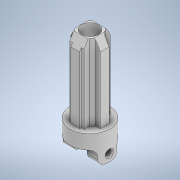
# Autodesk Inventor part: upper plug
Saved by Autodesk Inventor 2022 (Build 260153000, 153)
## iProperties
Created: 2022-03-20
Part Number: upper plug
Material: Generic
Document SubType Name: Modeling
Designer: Dahway
Density: 1 g/cm^3
Appearance: Default
Author: Dahway
Autodesk Inventor part; units mm, degrees
ref_plane "YZ Plane" through (0, 0, 0) normal (1, 0, 0) x (0, 1, 0)
ref_plane "XZ Plane" through (0, 0, 0) normal (0, 1, 0) x (-1, 0, 0)
ref_plane "XY Plane" through (0, 0, 0) normal (0, 0, 1) x (1, 0, 0)
sketch "Sketch1" plane through (0, 0, 0) normal (0, 1, 0) x (-1, 0, 0)
  circle A0 centre (0, 0) radius 7
  dimension "d0" = 14
  constraints: 1 centre point, 1 coincident
  measures "d0" diameter of A0
extrude "Extrusion1" add sketch "Sketch1" along normal blind 5
sketch "Sketch2" plane through (0, 5, 0) normal (0, 1, 0) x (1, 0, 0)
  circle A0 centre (0, 0) radius 3.8
  circle A1 centre (0, 0) radius 7 projected
  line L0 (-1.55, 5.2) -> (1.55, 5.2)
  line L1 (1.55, 5.2) -> (1.55, 2.4)
  line L2 (1.55, 2.4) -> (-1.55, 2.4)
  line L3 (-1.55, 2.4) -> (-1.55, 5.2)
  line L4 (-1.55, 5.2) -> (1.55, 2.4) construction
  line L5 (1.55, 5.2) -> (-1.55, 2.4) construction
  circle A2 centre (0, 0) radius 3.8
  line L6 (-5.2, -1.55) -> (-5.2, 1.55)
  line L7 (-5.2, 1.55) -> (-2.4, 1.55)
  line L8 (-2.4, 1.55) -> (-2.4, -1.55)
  line L9 (-2.4, -1.55) -> (-5.2, -1.55)
  line L10 (-5.2, -1.55) -> (-2.4, 1.55) construction
  line L11 (-5.2, 1.55) -> (-2.4, -1.55) construction
  circle A3 centre (0, 0) radius 3.8
  line L12 (1.55, -5.2) -> (-1.55, -5.2)
  line L13 (-1.55, -5.2) -> (-1.55, -2.4)
  line L14 (-1.55, -2.4) -> (1.55, -2.4)
  line L15 (1.55, -2.4) -> (1.55, -5.2)
  line L16 (1.55, -5.2) -> (-1.55, -2.4) construction
  line L17 (-1.55, -5.2) -> (1.55, -2.4) construction
  circle A4 centre (0, 0) radius 3.8
  line L18 (5.2, 1.55) -> (5.2, -1.55)
  line L19 (5.2, -1.55) -> (2.4, -1.55)
  line L20 (2.4, -1.55) -> (2.4, 1.55)
  line L21 (2.4, 1.55) -> (5.2, 1.55)
  line L22 (5.2, 1.55) -> (2.4, -1.55) construction
  line L23 (5.2, -1.55) -> (2.4, 1.55) construction
  line L24 (2.55, 4.6) -> (-2.55, 4.6)
  line L25 (-2.55, 4.6) -> (-2.55, 2.8174)
  line L26 (-2.55, 2.8174) -> (2.55, 2.8174)
  line L27 (2.55, 2.8174) -> (2.55, 4.6)
  line L28 (-2.55, -2.8174) -> (-2.55, -4.6)
  line L29 (-2.55, -4.6) -> (2.55, -4.6)
  line L30 (2.55, -4.6) -> (2.55, -2.8174)
  point P0 (0, 3.8)
  point P1 (-3.8, 0)
  point P2 (0, -3.8)
  point P3 (3.8, 0)
  point P4 (-1.55, 3.4695)
  point P5 (-3.4695, 1.55)
  point P6 (-3.4695, -1.55)
  point P7 (-1.55, -3.4695)
  point P8 (1.55, -3.4695)
  point P9 (3.4695, -1.55)
  point P10 (3.4695, 1.55)
  point P11 (1.55, 3.4695)
  point P12 (2.55, -2.8174)
  point P13 (1.55, -4.6)
  point P14 (-1.55, -4.6)
  point P15 (-2.55, -2.8174)
  point P16 (-2.55, 2.8174)
  point P17 (-1.55, 4.6)
  point P18 (2.55, 2.8174)
  point P19 (1.55, 4.6)
  dimension "d65" = 7.6
  dimension "d66" = 3.2
  dimension "d67" = 3.1
  dimension "d68" = 2.8
  dimension "d71" = 360
  dimension "d75" = 5.1
  dimension "d76" = 0.6
  dimension "d80" = 360
  dimension "d88" = 2.55
  dimension "d89" = 2.4
  constraints: 62 end point, 8 midpoint, 4 coincident, 4 parallel, 2 coincident with centre, 2 horizontal, 2 perpendicular, 2 point on circle, 1 centre point, 1 horizontal alignment, 1 vertical alignment, 71 other
  measures "d67" distance of L1.end L2.end
  measures "d68" distance of L0.end L1.end
  measures "d75" distance of L26.end L25.end
  measures "d76" distance between parallel lines of L24 L0
  measures "d88" distance from line of point (0, 0) L27
  measures "d89" distance from line of point (0, 0) L2
extrude "Extrusion2" add sketch "Sketch2" along normal blind 27 contours A0 L19 L20 L21 | A0 L21 L18 L19 | L21 L20 L19 A0 L15 L14 L13 L9 L8 L7 L26 L3 L2 L1 | L26 L1 A0 | A0 L1 L24 L27 | L30 L29 L15 A0 | L1 L26 L3 A0 | A0 L3 L24 L1 | L1 L2 L3 L26 | L15 L29 L13 A0 | A0 L13 L14 L15 | L3 L26 A0 | A0 L25 L24 L3 | L24 L3 L0 L1 | L13 L29 L28 A0 | L15 L12 L13 L29 | L7 L8 L9 A0 | A0 L9 L6 L7
sketch "Sketch3" plane through (0, 32, 0) normal (0, 1, 0) x (1, 0, 0)
  line L0 (-5.25, -1.5) -> (-3.4369, -1.5) projected
  line L1 (3.4369, -1.5) -> (5.25, -1.5) projected
  circle A0 centre (0, 0) radius 3
  point P0 (0, 0)
  dimension "d61" = 6
  constraints: 1 centre point, 1 coincident
  measures "d61" diameter of A0
extrude "Extrusion3" cut sketch "Sketch3" against normal blind 7
sketch "Sketch4" plane through (0, 5, 0) normal (0, 1, 0) x (1, 0, 0)
  circle A0 centre (0, 0) radius 7 projected
  line L0 (0, 0) -> (7, 0) construction
  line L1 (0, 0) -> (7, 0) construction
  circle A1 centre (-4.9497, 4.9497) radius 1
  circle A2 centre (-4.9497, -4.9497) radius 1
  circle A3 centre (4.9497, -4.9497) radius 1
  circle A4 centre (4.9497, 4.9497) radius 1
  point P0 (-4.9497, -4.9497)
  point P1 (4.9497, 4.9497)
  point P2 (4.1939, 5.6045)
  point P3 (5.6045, 4.1939)
  point P4 (5.6045, -4.1939)
  point P5 (4.1939, -5.6045)
  point P6 (-5.6045, -4.1939)
  point P7 (-4.1939, -5.6045)
  point P8 (-4.1939, 5.6045)
  point P9 (-5.6045, 4.1939)
  dimension "d26" = 2
  dimension "d29" = 360
  constraints: 4 centre point, 4 end point, 2 horizontal, 2 point on circle, 1 coincident, 9 other
  measures "d26" diameter of A1
extrude "Extrusion4" add sketch "Sketch4" along normal blind 2 contours A4 A0 | A0 A3 | A1 A0 | A0 A2 picked at (4.7103, 4.7103) picked at (4.7103, -4.7103) picked at (-4.6879, 4.735) picked at (-4.6879, -4.735)
sketch "Sketch5" plane through (0, 0, 0) normal (0, -1, 0) x (1, 0, 0)
  line L0 (2.5, 3.45) -> (2.5, -3.45)
  arc A0 (5.6045, -4.1939) -> (5.6045, 4.1939) centre (0, 0) ccw projected
  arc A1 (6.0908, -3.45) -> (6.0908, 3.45) centre (0, 0) ccw
  line L1 (2.5, 3.45) -> (6.0908, 3.45)
  line L2 (2.5, -3.45) -> (6.0908, -3.45)
  dimension "d33" = 6.9
  dimension "d50" = 4.5
  constraints: 6 end point, 4 point on circle, 2 parallel, 1 centre point, 1 horizontal, 1 vertical
  measures "d33" distance of L0.start L0.end
  measures "d50" distance edge to line of A0 L0
extrude "Extrusion5" add sketch "Sketch5" along normal blind 5
pattern_circular "Circular Pattern1" count 2 over 360 about axis through (0, 0, 0) along (0, 1, 0) of "Extrusion5"
fillet "Fillet2" radius 2 10 edges at (4.2954, -5, -3.45) (4.2954, -5, 3.45) (-4.2954, -5, -3.45) (-4.2954, -5, 3.45) (4.2954, 0, -3.45) (-4.2954, 0, -3.45) (-4.2954, 0, 3.45) (4.2954, 0, 3.45) (2.5, 0, 0) (-2.5, 0, 0)
sketch "Sketch7" plane through (2.5, -3, -3.45) normal (-1, 0, 0) x (0, 0, 1)
  line L0 (4.9, -2) -> (2, -2) projected
  line L1 (0, 1) -> (0, 0) projected
  point P0 (3.45, 3)
  point P1 (3.45, 0.5)
  dimension "d52" = 2.5
  dimension "d53" = 3.45
  measures "d52" distance from line of L0 point (3.45, 0.5)
  measures "d53" distance from line of point (3.45, 0.5) L1
hole "Hole2" at (2.5, -2.5, 0) direction (1, 0, 0) diameter 2 end through all both
chamfer "Chamfer2" distance 0.5 angle 45 8 edges at (6.9282, -2.5039, -1) (-6.9282, -2.5039, -1) (2.5, -2.2412, 0.9659) (2.5, -3.4659, -0.2588) (2.4365, -1.5, 0) (-2.5, -3.4659, -0.2588) (-2.5, -2.2412, 0.9659) (-2.4365, -1.5, 0)
chamfer "Chamfer3" distance 2 angle 60 4 edges at (5.2, 32, 0) (0, 32, -5.2) (-5.2, 32, 0) (0, 32, 5.2) measured on face at (0, 32, 4.7) measured on face at (0, 32, -4.7) measured on face at (-4.7, 32, 0) measured on face at (4.7, 32, 0)
sketch "Sketch9" plane through (0, 5, 0) normal (0, 1, 0) x (1, 0, 0)
  arc A0 (-4.1939, -5.6045) -> (-5.6045, -4.1939) centre (-4.9497, -4.9497) ccw projected
  circle A1 centre (-4.9497, -4.9497) radius 1
  arc A2 (5.6045, -4.1939) -> (4.1939, -5.6045) centre (4.9497, -4.9497) ccw projected
  circle A3 centre (4.9497, -4.9497) radius 1
  arc A4 (4.1939, 5.6045) -> (5.6045, 4.1939) centre (4.9497, 4.9497) ccw projected
  circle A5 centre (4.9497, 4.9497) radius 1
  circle A6 centre (-4.9497, 4.9497) radius 1
  point P0 (0, 0)
  point P1 (-5.6045, -4.1939)
  point P2 (5.6045, 4.1939)
  point P3 (4.1939, 5.6045)
  point P4 (4.1939, -5.6045)
  constraints: 4 centre point, 3 coincident
extrude "Extrusion6" cut sketch "Sketch9" along normal up to surface (2 mm away)
body "Solid1"
